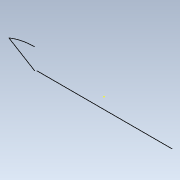
# Autodesk Inventor part: acrlyc 2.0
Saved by Autodesk Inventor 2021 (Build 250183000, 183)
## iProperties
Created: 2020-10-01
Part Number: acrlyc 2.0
Material: Generic
Document SubType Name: Modeling
Designer: capta
Density: 1 g/cm^3
Appearance: Default
Author: capta
Autodesk Inventor part; units mm, degrees
ref_plane "YZ Plane" through (0, 0, 0) normal (1, 0, 0) x (0, 1, 0)
ref_plane "XZ Plane" through (0, 0, 0) normal (0, 1, 0) x (-1, 0, 0)
ref_plane "XY Plane" through (0, 0, 0) normal (0, 0, 1) x (1, 0, 0)
sketch "Sketch1" plane through (0, 0, 0) normal (0, 0, 1) x (1, 0, 0)
  line L0 (-7.4316, -27.4282) -> (-35.2065, -10.3786)
  ellipse E0 centre (-9.4295, -71.0975) end of major axis (56.853, -71.097) minor radius 65.907 (-9.4295, -5.1905) -> (-35.2065, -10.3786) ccw
  line L1 (-9.4295, -5.1905) -> (130.2705, -5.1905)
  ellipse E1 centre (130.2705, -71.0975) end of major axis (196.553, -71.0979) minor radius 65.907 (156.0476, -10.3786) -> (130.2705, -5.1905) ccw
  line L2 (156.0476, -10.3786) -> (128.2727, -27.4282)
  line L3 (128.2727, -27.4282) -> (-7.4316, -27.4282)
  constraints: 8 end point, 2 horizontal, 18 other
extrude "Extrusion1" add sketch "Sketch1" along normal blind 1.27
body "Solid1"
